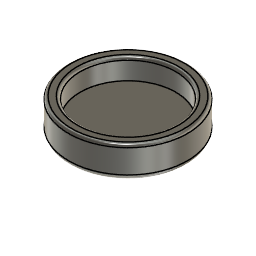
Magnet Holder_v5 (Autodesk Fusion 360 design; units mm, degrees)
Autodesk Fusion 360 part; units mm, degrees
sketch "Sketch1" plane through (0, 0, 0) normal (0, 0, 1) x (1, 0, 0)
  circle A0 centre (0, 0) radius 4.1
  circle A1 centre (0, 0) radius 5.1
  circle A2 centre (-2.3, 0) radius 1.5
  dimension "d1" = 8.2
  dimension "d2" = 1
  dimension "d12" = 3
  constraint coincident A0.centre A1.centre
  measures "d1" diameter of A0
  measures "d2" distance of A0 A1
  measures "d12" diameter of A2
extrude "Extrude1" add sketch "Sketch1" along normal blind 1 contours A0 | A1 | A2
extrude "Extrude2" add sketch "Sketch1" along normal blind 2.775 contours A1
fillet "Fillet1" radius 0.25 2 edges at (-3.8225, 1.4826, 2.775) (-4.7549, -1.8442, 2.775)
extrude "Extrude3" add sketch "Sketch1" against normal blind 2 contours A2
fillet "Fillet2" radius 0.5 1 edges at (-4.7549, -1.8442, 0)
move_face "OffsetFaces1" offset 0.2 1 faces at (-0.8019, -0.0748, -1.3333)
chamfer "Chamfer1" distance 2 distance2 0.1 1 faces at (-0.6021, -0.0847, -1.3333) tangent chain off
equation "d5 = 1 mm + 1.775 mm"
